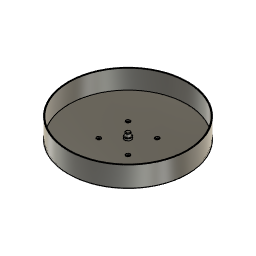
Turntable Spool holder Lid v3 (Autodesk Fusion 360 design; units mm, degrees)
Autodesk Fusion 360 part; units mm, degrees
note: some values were not read from the file. Set by a fixed rule: which sketch regions a step uses.
sketch "Sketch1" plane through (0, 0, 0) normal (0, 0, 1) x (1, 0, 0)
  circle A0 centre (0, 0) radius 5.75
  circle A1 centre (0, 0) radius 100.75
  circle A2 centre (0, 0) radius 3.975
  circle A3 centre (0, 0) radius 102.25
  line L0 (-25, -25) -> (25, -25)
  line L1 (25, -25) -> (25, 25)
  line L2 (25, 25) -> (-25, 25)
  line L3 (-25, 25) -> (-25, -25)
  line L4 (-25, -25) -> (25, 25) construction
  line L5 (25, -25) -> (-25, 25) construction
  circle A4 centre (25, -25) radius 3.5
  circle A5 centre (-25, -25) radius 3.5
  circle A6 centre (25, 25) radius 3.5
  circle A7 centre (-25, 25) radius 3.5
  circle A8 centre (-25, -25) radius 1.75
  circle A9 centre (-25, 25) radius 1.75
  circle A10 centre (25, 25) radius 1.75
  circle A11 centre (25, -25) radius 1.75
  dimension "d1" = 11.5
  dimension "d2" = 201.5
  dimension "d3" = 7.95
  dimension "d11" = 204.5
  dimension "d24" = 50
  dimension "d25" = 50
  dimension "d26" = 7
  dimension "d27" = 7
  dimension "d28" = 7
  dimension "d29" = 7
  dimension "d30" = 3.5
  dimension "d31" = 3.5
  dimension "d32" = 3.5
  dimension "d33" = 3.5
  constraint coincident A0.centre A1.centre
  constraint concentric A0 A1
  constraint concentric A0 A2
  constraint horizontal L0
  constraint perpendicular L0 L1
  constraint parallel L0 L2
  constraint parallel L1 L3
  constraint coincident L4 A0.centre
  constraint coincident L5 A0.centre
  constraint coincident L0.end L1.start
  constraint coincident L0.start L3.end
  constraint coincident L1.end L2.start
  constraint coincident L2.end L3.start
  constraint concentric A5 A8
  constraint concentric A7 A9
  constraint concentric A6 A10
  constraint concentric A4 A11
  measures "d1" diameter of A0
  measures "d2" diameter of A1
  measures "d3" diameter of A2
  measures "d11" diameter of A3
  measures "d24" distance of L1.end L2.end
  measures "d25" distance of L0.end L1.end
  measures "d26" diameter of A4
  measures "d27" diameter of A5
  measures "d28" diameter of A6
  measures "d29" diameter of A7
  measures "d30" diameter of A8
  measures "d31" diameter of A9
  measures "d32" diameter of A10
  measures "d33" diameter of A11
extrude "Extrude1" add sketch "Sketch1" along normal blind 6.5 contours A2
extrude "Extrude2" add sketch "Sketch1" against normal blind 3 contours A0 | A2
extrude "Extrude3" add sketch "Sketch1" against normal blind 3 from surface at -3 contours A0 | A1 | A2 | L0 L3 A8 | L0 L3 A8 | L0 L3 A5 A8 | L0 L3 A5 A8 | L0 L1 L2 L3 A4 A5 A6 A7 | L0 L1 A4 A11 | L0 L1 A4 A11 | L2 L3 A7 A9 | L2 L3 A7 A9 | L0 L1 A11 | L0 L1 A11 | L2 L3 A9 | L2 L3 A9 | L1 L2 A6 A10 | L1 L2 A6 A10 | L1 L2 A10 | L1 L2 A10
extrude "Extrude4" add sketch "Sketch1" along normal blind 68 from surface at -6 contours A3
chamfer "Chamfer1" distance 1 angle 45 1 edges at (-3.706, -1.4374, 6.5)
chamfer "Chamfer2" distance 0.5 angle 45 2 edges at (-95.3305, -36.9752, 62) (-93.932, 36.4328, 62)
chamfer "Chamfer3" distance 1 angle 45 1 edges at (-95.3305, -36.9752, -6)
extrude "Extrude6" cut sketch "Sketch1" against normal blind 15 contours L0 L3 A8 | L0 L3 A8 | L0 L1 A11 | L0 L1 A11 | L2 L3 A9 | L2 L3 A9 | L1 L2 A10 | L1 L2 A10
extrude "Extrude7" cut sketch "Sketch1" against normal blind 5 contours L0 L3 A5 A8 | L0 L3 A5 A8 | L0 L1 A4 A11 | L0 L1 A4 A11 | L2 L3 A7 A9 | L2 L3 A7 A9 | L1 L2 A6 A10 | L1 L2 A6 A10
extrude "Extrude9" cut sketch "Sketch1" along normal blind 45 from surface at 30 contours A3
chamfer "Chamfer4" distance 0.5 angle 45 2 edges at (-93.932, -36.4328, 30) (-95.3305, 36.9752, 30)
